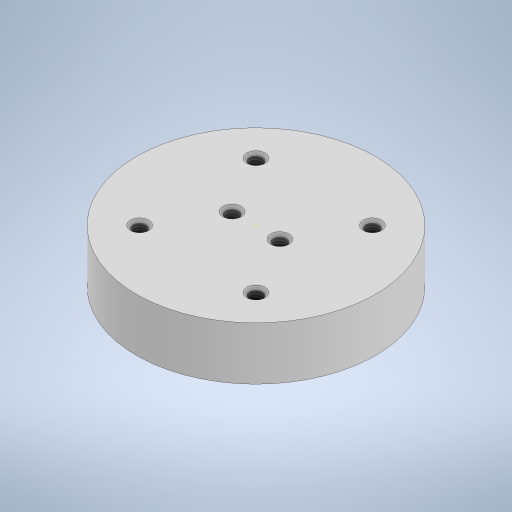
# Autodesk Inventor part: Диск (маховик, вал)
Saved by Autodesk Inventor 2023 (Build 270158000, 158)
## iProperties
Created: 2022-05-01
Part Number: Диск (маховик, вал)
Material: Типовые
Document SubType Name: Modeling
Designer: User
Density: 1 g/cm^3
Appearance: По умолчанию
Author: User
Autodesk Inventor part; units mm, degrees
ref_plane "YZ Plane" through (0, 0, 0) normal (1, 0, 0) x (0, 1, 0)
ref_plane "XZ Plane" through (0, 0, 0) normal (0, 1, 0) x (-1, 0, 0)
ref_plane "XY Plane" through (0, 0, 0) normal (0, 0, 1) x (1, 0, 0)
sketch "Эскиз1" plane through (0, 0, 0) normal (0, 1, 0) x (-1, 0, 0)
  circle A0 centre (0, 0) radius 22.5
  dimension "d0" = 45
  constraints: 1 centre point, 1 coincident
  measures "d0" diameter of A0
extrude "Выдавливание1" add sketch "Эскиз1" along normal blind 10
sketch "Эскиз2" plane through (0, 10, 0) normal (0, 1, 0) x (1, 0, 0)
  line L0 (0, 0) -> (-4.5, 0)
  line L1 (-4.5, 0) -> (4.5, 0)
  dimension "d3" = 4.5
  dimension "d4" = 9
  constraints: 4 end point, 1 horizontal, 1 point on line
  measures "d3" distance of L0.start L0.end
  measures "d4" distance of L0.end L1.end
hole "Отверстие1" at (-4.5, 10, 0) at (4.5, 10, 0) direction (0, -1, 0) diameter 2.459 end through all thread size "M3x0.5" class "6H" standard "ISO Metric profile"
sketch "Эскиз3" plane through (0, 10, 0) normal (0, 1, 0) x (1, 0, 0)
  point P0 (0, 0)
sketch "Эскиз4" plane through (0, 0, 0) normal (0, -1, 0) x (1, 0, 0)
  circle A0 centre (0, 0) radius 15.5
  line L0 (15.5, 15.5) -> (-15.5, 15.5)
  line L1 (-15.5, 15.5) -> (-15.5, -15.5)
  line L2 (-15.5, -15.5) -> (15.5, -15.5)
  line L3 (15.5, -15.5) -> (15.5, 15.5)
  line L4 (15.5, 15.5) -> (-15.5, -15.5)
  line L5 (15.5, -15.5) -> (-15.5, 15.5)
  point P0 (10.9602, 10.9602)
  point P1 (-10.9602, 10.9602)
  point P2 (-10.9602, -10.9602)
  point P3 (10.9602, -10.9602)
  dimension "d12" = 31
  constraints: 12 end point, 4 point on circle, 4 point on line, 2 parallel, 2 perpendicular, 1 centre point, 1 coincident, 1 horizontal
  measures "d12" diameter of A0
hole "Отверстие2" at (10.9602, 0, -10.9602) at (-10.9602, 0, -10.9602) at (-10.9602, 0, 10.9602) at (10.9602, 0, 10.9602) direction (0, 1, 0) diameter 2.459 end through all thread size "M3x0.5" class "6H" standard "ISO Metric profile"
chamfer "Фаска1" distance 0.5 angle 45 12 edges at (10.9602, 0, 12.1897) (10.9602, 0, -9.7307) (4.5, 0, -1.2295) (-4.5, 0, -1.2295) (-10.9602, 0, -9.7307) (-10.9602, 0, 12.1897) (10.9602, 10, -9.7307) (-10.9602, 10, -9.7307) (-4.5, 10, -1.2295) (4.5, 10, -1.2295) (10.9602, 10, 12.1897) (-10.9602, 10, 12.1897)
